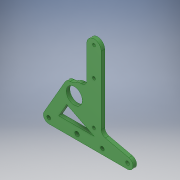
# Autodesk Inventor part: support plate
Saved by Autodesk Inventor 2017 SP1 (Build 210196100, 196)
## iProperties
Created: 2018-02-02
Part Number: support plate
Material: Generic
Document SubType Name: Modeling
Designer: Ben
Density: 1 g/cm^3
Appearance: Smooth - Dark Forest Green
Author: Ben
Autodesk Inventor part; units mm, degrees
ref_plane "YZ Plane" through (0, 0, 0) normal (1, 0, 0) x (0, 1, 0)
ref_plane "XZ Plane" through (0, 0, 0) normal (0, 1, 0) x (-1, 0, 0)
ref_plane "XY Plane" through (0, 0, 0) normal (0, 0, 1) x (1, 0, 0)
sketch "0" plane through (0, 0, 0) normal (0, 0, 1) x (1, 0, 0)
  line L0 (0, -12.7) -> (-62.4677, -12.7)
  line L1 (-62.4677, -12.7) -> (-48.3452, 11.8585)
  line L2 (-48.3452, 11.8585) -> (0, -12.7)
  line L3 (12.7, 3.512) -> (12.7, 123.825)
  arc A0 (12.7, 123.825) -> (-12.7, 123.825) centre (0, 123.825) ccw
  line L4 (-12.7, 123.825) -> (-12.7, 66.2826)
  arc A1 (-22.225, 56.7576) -> (-12.7, 66.2826) centre (-22.225, 66.2826) ccw
  arc A2 (-22.225, 56.7576) -> (-32.1229, 53.5191) centre (-22.225, 40.0127) ccw
  arc A3 (-42.0209, 50.2806) -> (-32.1229, 53.5191) centre (-42.0209, 67.0256) ccw
  arc A4 (-42.0209, 50.2806) -> (-51.3186, 44.9019) centre (-42.0209, 39.5552) ccw
  line L5 (-51.3186, 44.9019) -> (-88.3941, -19.5709)
  arc A5 (-88.3941, -19.5709) -> (-80.137, -33.8442) centre (-80.137, -24.3192) ccw
  line L6 (-80.137, -33.8442) -> (59.563, -33.8442)
  arc A6 (59.563, -33.8442) -> (61.6718, -15.0305) centre (59.563, -24.3192) ccw
  line L7 (61.6718, -15.0305) -> (19.9403, -5.5562)
  arc A7 (12.7, 3.512) -> (19.9403, -5.5562) centre (21.999, 3.512) ccw
  circle A8 centre (0, 0) radius 2.667
  circle A9 centre (0, 76.2) radius 2.667
  circle A10 centre (0, 127) radius 2.667
  circle A11 centre (59.563, -24.3192) radius 3.3528
  circle A12 centre (14.7822, -24.3192) radius 3.3528
  circle A13 centre (-80.137, -24.3192) radius 3.3528
  circle A14 centre (-30, -24.3192) radius 4.064
  circle A15 centre (-34.925, 31.75) radius 14.2875
  line L8 (0, 127) -> (0, 0) construction
  line L9 (-80.137, -24.3192) -> (14.7822, -24.3192) construction
  line L10 (14.7822, -24.3192) -> (59.563, -24.3192) construction
  line L11 (-84.4429, -12.7) -> (51.4065, -12.7) construction
  line L12 (-22.225, 56.7576) -> (0, 56.7576) construction
  line L13 (-42.0209, 50.2806) -> (0, 50.2806) construction
  line L14 (-52.9282, 42.1029) -> (-47.3106, 38.8724) construction
  line L15 (-45.7096, 10.5197) -> (-41.3958, 19.0118) construction
  dimension "d0" = 5.334
  dimension "d1" = 76.2
  dimension "d2" = 127
  dimension "d3" = 12.7
  dimension "d4" = 3.175
  dimension "d5" = 6.7056
  dimension "d6" = 28.575
  dimension "d8" = 12.7
  dimension "d9" = 12.7
  dimension "d10" = 9.525
  dimension "d11" = 10.7254
  dimension "d12" = 56.7576
  dimension "d13" = 6.477
  dimension "d14" = 34.925
  dimension "d15" = 44.45
  dimension "d16" = 6.4802
  dimension "d17" = 50.137
  dimension "d18" = 44.7822
  dimension "d19" = 44.7808
  dimension "d22" = 11.6192
  dimension "d23" = 8.128
  dimension "d24" = 59.563
  dimension "d25" = 9.525
  dimension "d26" = 9.299
  dimension "d27" = 16.212
  dimension "d28" = 19.05
  dimension "d29" = 9.525
  constraints: 32 end point, 18 point on circle, 16 centre point, 14 tangent, 12 point on line, 6 equal radius, 4 perpendicular, 3 coincident, 2 horizontal, 2 parallel, 2 vertical, 1 collinear
  measures "d0" diameter of A8
  measures "d1" distance of L8.end A9.centre
  measures "d2" distance of L8.start L8.end
  measures "d3" radius of A0
  measures "d4" distance of L8.start A0.centre
  measures "d5" diameter of A11
  measures "d6" diameter of A15
  measures "d8" distance from line of L8.end L11
  measures "d9" distance between parallel lines of L8 L3
  measures "d10" radius of A1
  measures "d11" radius of A4
  measures "d12" distance from line of L8.end L12
  measures "d13" distance between parallel lines of L13 L12
  measures "d14" distance from line of L8 A15.centre
  measures "d15" distance from line of L11 A15.centre
  measures "d16" distance of L14.start L14.end
  measures "d17" distance of L9.start A14.centre
  measures "d18" distance of L9.end A14.centre
  measures "d19" distance of A6.centre L9.end
  measures "d22" distance from line of A14.centre L11
  measures "d23" diameter of A14
  measures "d24" horizontal distance of L10.end L8.end
  measures "d25" radius of A6
  measures "d26" radius of A7
  measures "d27" distance from line of L11 L3.start
  measures "d28" distance between parallel lines of L5 L1
  measures "d29" distance of L15.start L15.end
extrude "Extrusion1" add sketch "0" along normal blind 6.35
chamfer "Chamfer1" distance 2.3813 angle 45 3 edges at (-2.667, 127, 0) (-2.667, 76.2, 0) (-2.667, 0, 0)
body "Solid1"
